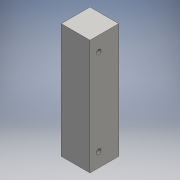
# Autodesk Inventor part: Blok_roda
Saved by Autodesk Inventor 2016 SP2 (Build 200236200, 236)
## iProperties
Created: 2017-09-11
Part Number: Blok_roda
Material: Generic
Document SubType Name: Modeling
Designer: Admin
Density: 1 g/cm^3
Appearance: Default
Author: Admin
Autodesk Inventor part; units mm, degrees
ref_plane "YZ Plane" through (0, 0, 0) normal (1, 0, 0) x (0, 1, 0)
ref_plane "XZ Plane" through (0, 0, 0) normal (0, 1, 0) x (-1, 0, 0)
ref_plane "XY Plane" through (0, 0, 0) normal (0, 0, 1) x (1, 0, 0)
sketch "Sketch1" plane through (0, 0, 0) normal (0, 0, 1) x (1, 0, 0)
  line L0 (25, -25) -> (-25, -25)
  line L1 (-25, -25) -> (-25, 25)
  line L2 (-25, 25) -> (25, 25)
  line L3 (25, 25) -> (25, -25)
  line L4 (25, -25) -> (-25, 25) construction
  line L5 (-25, -25) -> (25, 25) construction
  point P0 (0, 0)
  dimension "d0" = 50
  dimension "d1" = 50
  constraints: 12 end point, 2 midpoint, 2 parallel, 1 horizontal, 1 perpendicular
  measures "d0" distance of L1.end L2.end
  measures "d1" distance of L0.end L1.end
extrude "Extrusion1" add sketch "Sketch1" along normal blind 200
sketch "Sketch2" plane through (25, -25, 0) normal (1, 0, 0) x (0, 0, -1)
  circle A0 centre (-175, 15) radius 4
  circle A1 centre (-25, 15) radius 4
  line L0 (0, 0) -> (-200, 0) projected
  line L1 (-200, 0) -> (-200, 50) projected
  point P0 (0, 25)
  dimension "d4" = 8
  dimension "d5" = 15
  dimension "d6" = 8
  dimension "d7" = 15
  dimension "d8" = 25
  dimension "d9" = 25
  constraints: 2 centre point
  measures "d4" diameter of A0
  measures "d5" vertical distance of L0.end A0.centre
  measures "d6" diameter of A1
  measures "d7" distance from line of L0 A1.centre
  measures "d8" distance from line of L1 A0.centre
  measures "d9" horizontal distance of point (0, 25) A1.centre
extrude "Extrusion2" cut sketch "Sketch2" against normal through all
body "Solid1"
